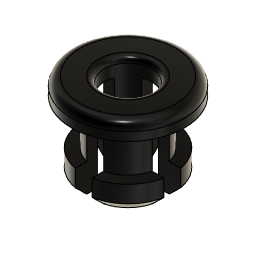
Valkyrie Filament ROS (Autodesk Fusion 360 archive; units mm, degrees)
design "Tube Collet"
Autodesk Fusion 360 part; units mm, degrees
sketch "Sketch1" plane through (0, 0, 0) normal (1, 0, 0) x (0, 1, 0)
  line L0 (0, 0) -> (0, 8)
  line L1 (0, 8) -> (5, 8)
  line L2 (5, 8) -> (5, 6.5)
  line L3 (5, 6.5) -> (3, 6.5)
  line L4 (3, 6.5) -> (3, 2.5)
  line L5 (0, 0) -> (4, 0)
  line L6 (4, 0) -> (4, 2.5)
  line L7 (4, 2.5) -> (3, 2.5)
  dimension "d7000" = 1.5
  dimension "d7001" = 2.5
  dimension "d7002" = 8
  dimension "d7003" = 4
  dimension "d7004" = 6
  dimension "d7005" = 10
  dimension "d7006" = 8
  constraint coincident L0.start L5.start
  constraint vertical L0
  constraint horizontal L1
  constraint vertical L2
  constraint horizontal L3
  constraint vertical L4
  constraint horizontal L5
  constraint vertical L6
  constraint horizontal L7
  constraint coincident L4.end L7
  measures "d7000" distance of L1.end L2.end
  measures "d7001" distance of L5.end L6.end
  measures "d7002" distance of L0.start L0.end
  measures "d7003" distance of L3.end L4.end
revolve "Revolve1" add sketch "Sketch1" angle 360 about axis through (0, 0, 0) along (0, 0, 1)
hole "Hole1" at (0, 0, 8) direction (0, 0, -1) diameter 4.2 depth 10.5 tip angle 118
chamfer "Chamfer1" distance 1 angle 45 1 edges at (-3.7293, 1.4465, 0)
sketch "Sketch2" plane through (0, 0, 0) normal (0, 0, -1) x (1, 0, 0)
  circle A0 centre (0, 0) radius 2.1
  circle A1 centre (0, 0) radius 3
  circle A2 centre (0, 0) radius 4
  circle A3 centre (0, 0) radius 3
  line L0 (4, -0.75) -> (-4, -0.75)
  line L1 (-4, -0.75) -> (-4, 0.75)
  line L2 (-4, 0.75) -> (4, 0.75)
  line L3 (4, 0.75) -> (4, -0.75)
  line L4 (4, -0.75) -> (-4, 0.75) construction
  line L5 (-4, -0.75) -> (4, 0.75) construction
  line L6 (-0.75, 4) -> (0.75, 4)
  line L7 (0.75, 4) -> (0.75, -4)
  line L8 (0.75, -4) -> (-0.75, -4)
  line L9 (-0.75, -4) -> (-0.75, 4)
  line L10 (-0.75, 4) -> (0.75, -4) construction
  line L11 (0.75, 4) -> (-0.75, -4) construction
  dimension "d7012" = 1.5
  dimension "d7013" = 1.5
  constraint horizontal L0
  constraint perpendicular L0 L1
  constraint parallel L0 L2
  constraint parallel L1 L3
  constraint coincident L4 A0.centre
  constraint coincident L5 A0.centre
  constraint coincident A0.centre A1.centre
  constraint tangent A2 L3
  constraint horizontal L6
  constraint perpendicular L6 L7
  constraint parallel L6 L8
  constraint parallel L7 L9
  constraint coincident L10 A0.centre
  constraint coincident L11 A0.centre
  constraint tangent A2 L6
  measures "d7012" distance of L0.start L2.end
  measures "d7013" distance of L6.start L6.end
extrude "Extrude1" cut sketch "Sketch2" against normal up to surface (6.5 mm away) contours A0 L0 L2 L7 | A0 A1 A3 L0 L2 | A0 L2 L7 L9 | A0 A1 A3 L7 L9 | L0 L2 L7 L9 | A1 A2 A3 L0 L2 | A0 A1 A3 L7 L9 | A0 L0 L7 L9 | A1 A2 A3 L7 L9 | A0 L0 L2 L9 | A1 A2 A3 L7 L9 | A0 A1 A3 L0 L2 | A1 A2 A3 L0 L2
fillet "Fillet1" radius 0.75 1 edges at (-4.6616, 1.8081, 8)
fillet "Fillet1" radius 0.5 1 edges at (-1.9579, 0.7594, 8)
